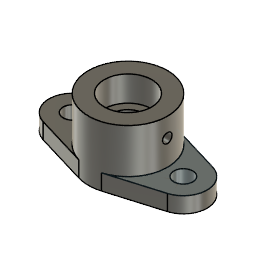
8- CUT SECTION OF SOLIDS (Autodesk Fusion 360 design; units mm, degrees)
part number: 2026-02-24-15-10-40-431
Autodesk Fusion 360 part; units mm, degrees
sketch "Sketch1" plane through (0, 0, 0) normal (0, 0, 1) x (1, 0, 0)
  circle A0 centre (-35, 0) radius 6
  circle A1 centre (35, 0) radius 6
  line L0 (-39.2857, 14.3747) -> (-7.1429, 23.9579)
  line L1 (-39.2857, -14.3747) -> (-7.1429, -23.9579)
  line L2 (7.1429, 23.9579) -> (39.2857, 14.3747)
  line L3 (7.1429, -23.9579) -> (39.2857, -14.3747)
  arc A2 (39.2857, -14.3747) -> (39.2857, 14.3747) centre (35, 0) ccw
  arc A3 (-39.2857, 14.3747) -> (-39.2857, -14.3747) centre (-35, 0) ccw
  arc A4 (-7.1429, -23.9579) -> (7.1429, -23.9579) centre (0, 0) ccw
  arc A5 (7.1429, 23.9579) -> (-7.1429, 23.9579) centre (0, 0) ccw
  dimension "d3" = 50
  dimension "d4" = 12
  dimension "d5" = 12
  dimension "d6" = 35
  dimension "d7" = 35
  dimension "d8" = 30
  dimension "d9" = 30
  constraint coincident A4.centre A5.centre
  constraint concentric A0 A3
  constraint concentric A1 A2
  constraint tangent L0 A3
  constraint tangent L0 A5
  constraint tangent L1 A3
  constraint tangent L1 A4
  constraint tangent L2 A5
  constraint tangent L2 A2
  constraint tangent L3 A4
  constraint tangent L3 A2
  constraint concentric A4 A5
  measures "d3" diameter of A4
  measures "d4" diameter of A0
  measures "d5" diameter of A1
  measures "d6" distance of A4.centre A0.centre
  measures "d7" distance of A4.centre A1.centre
  measures "d8" diameter of A3
  measures "d9" diameter of A2
extrude "Extrude1" add sketch "Sketch1" along normal blind 10
sketch "Sketch2" plane through (0, 0, 10) normal (0, 0, 1) x (-1, 0, 0)
  circle A0 centre (-35, 0) radius 6
  circle A1 centre (35, 0) radius 6
  arc A2 (39.2857, -14.3747) -> (39.2857, 14.3747) centre (35, 0) ccw
  line L0 (39.2857, 14.3747) -> (7.1429, 23.9579)
  arc A3 (7.1429, 23.9579) -> (-7.1429, 23.9579) centre (0, 0) ccw
  line L1 (-7.1429, 23.9579) -> (-39.2857, 14.3747)
  arc A4 (-39.2857, 14.3747) -> (-39.2857, -14.3747) centre (-35, 0) ccw
  line L2 (-39.2857, -14.3747) -> (-7.1429, -23.9579)
  arc A5 (-7.1429, -23.9579) -> (7.1429, -23.9579) centre (0, 0) ccw
  line L3 (7.1429, -23.9579) -> (39.2857, -14.3747)
  circle A6 centre (0, 0) radius 25
  circle A7 centre (0, 0) radius 15
  circle A8 centre (0, 0) radius 10
  dimension "d12" = 50
  dimension "d13" = 30
  dimension "d14" = 20
  constraint coincident A3.centre A5.centre
  constraint concentric A6 A7
  constraint concentric A7 A8
  measures "d12" diameter of A6
  measures "d13" diameter of A7
  measures "d14" diameter of A8
extrude "Extrude2" add sketch "Sketch2" along normal blind 28 contours A3 A5 A6
sketch "Sketch3" plane through (0, 0, 10) normal (0, 0, 1) x (-1, 0, 0)
  circle A0 centre (0, 0) radius 15
  circle A1 centre (0, 0) radius 10
  dimension "d17" = 20
  constraint coincident A0.centre A1.centre
  measures "d17" diameter of A1
extrude "Extrude3" add sketch "Sketch3" along normal blind 12
sketch "Sketch4" plane through (0, 0, 10) normal (0, 0, 1) x (-1, 0, 0)
  circle A0 centre (-35, 0) radius 6
  arc A1 (-7.1429, 23.9579) -> (-7.1429, -23.9579) centre (0, 0) ccw
  line L0 (-7.1429, 23.9579) -> (-39.2857, 14.3747)
  arc A2 (-39.2857, 14.3747) -> (-39.2857, -14.3747) centre (-35, 0) ccw
  line L1 (-39.2857, -14.3747) -> (-7.1429, -23.9579)
sketch "Sketch5" plane through (0, 0, 0) normal (1, 0, 0) x (0, 1, 0)
  circle A0 centre (0, 26) radius 3
  line L0 (25, 38) -> (-25, 38)
  dimension "d20" = 6
  dimension "d21" = 12
  measures "d20" diameter of A0
  measures "d21" distance of A0.centre L0
extrude "Extrude4" cut sketch "Sketch5" along normal blind 25
sketch "Sketch6" plane through (0, 0, 0) normal (1, 0, 0) x (0, 1, 0)
